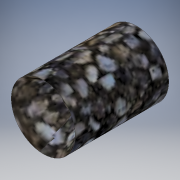
# Autodesk Inventor part: optimum nozzle
Saved by Autodesk Inventor 2019 (Build 230136000, 136)
## iProperties
Created: 2021-04-26
Part Number: optimum nozzle
Material: Concrete
Document SubType Name: Modeling
Designer: Mike
Density: 2.40731 g/cm^3
Appearance: Exposed Aggregate - Coarse
Author: Mike
Autodesk Inventor part; units mm, degrees
ref_plane "YZ Plane" through (0, 0, 0) normal (1, 0, 0) x (0, 1, 0)
ref_plane "XZ Plane" through (0, 0, 0) normal (0, 1, 0) x (-1, 0, 0)
ref_plane "XY Plane" through (0, 0, 0) normal (0, 0, 1) x (1, 0, 0)
sketch "Sketch1" plane through (0, 0, 0) normal (1, 0, 0) x (0, 1, 0)
  line L0 (0, 0) -> (15.5, 0)
  line L1 (15.5, 0) -> (35.6424, 0) construction
  line L2 (0, 0) -> (5.5, 0)
  line L3 (15.5, 0) -> (5.5, -14.2815)
  line L4 (15.5, 0) -> (45.1831, 0) construction
  line L5 (5.5, -14.2815) -> (5.5, -19.2815)
  line L6 (5.5, -19.2815) -> (11, -45.1569)
  line L7 (0, 0) -> (11, 0)
  line L8 (15.5, 0) -> (5.5, 0)
  line L9 (11, -45.1569) -> (5.5, -45.1569)
  line L10 (15.5, 0) -> (15.5, -45.1569)
  line L11 (15.5, -45.1569) -> (11, -45.1569)
  line L12 (0, -54.1883) -> (0, 9.0314) projected
  dimension "d0" = 15.5
  dimension "d3" = 5.5
  dimension "d4" = 125
  dimension "d6" = 5
  dimension "d7" = 168
  dimension "d8" = 11
  dimension "d9" = 45.157
  dimension "d10" = 25.8755
  dimension "d11" = 45.157
  constraints: 24 end point, 3 horizontal, 3 point on line, 1 collinear, 1 perpendicular, 1 vertical
  measures "d0" distance of L0.start L0.end
  measures "d3" distance of L0.start L2.end
  measures "d4" angle of L3 L4
  measures "d6" distance of L3.end L5.end
  measures "d7" angle of L6 L5
  measures "d8" distance of L0.start L7.end
  measures "d9" vertical distance of L6.end L0.start
  measures "d10" vertical distance of L6.end L5.end
  measures "d11" distance of L10.end L0.end
revolve "Revolution1" add sketch "Sketch1" angle 360 about axis through (0, 0, -10) along (0, 0, 1)
body "Solid1"
